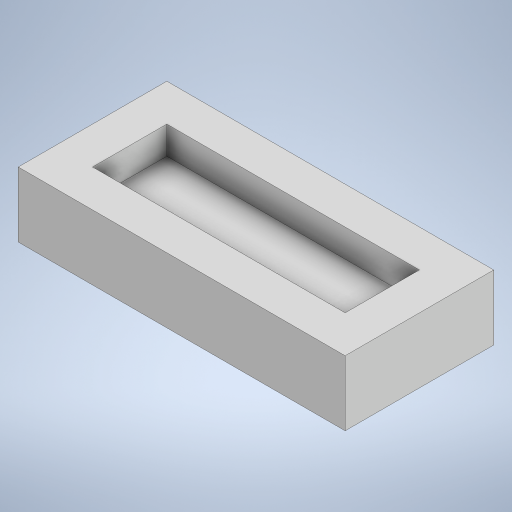
# Autodesk Inventor part: Connector Cover
Saved by Autodesk Inventor 2024 (Build 280153000, 153)
## iProperties
Created: 2023-09-15
Part Number: Connector Cover
Material: Generic
Document SubType Name: Modeling
Designer: cfang
Density: 1 g/cm^3
Appearance: Default
Author: cfang
Autodesk Inventor part; units mm, degrees
ref_plane "YZ Plane" through (0, 0, 0) normal (1, 0, 0) x (0, 1, 0)
ref_plane "XZ Plane" through (0, 0, 0) normal (0, 1, 0) x (-1, 0, 0)
ref_plane "XY Plane" through (0, 0, 0) normal (0, 0, 1) x (1, 0, 0)
sketch "Sketch1" plane through (0, 0, 0) normal (0, 1, 0) x (-1, 0, 0)
  line L0 (-8.8, -4) -> (8.8, -4)
  line L1 (8.8, -4) -> (8.8, 4)
  line L2 (8.8, 4) -> (-8.8, 4)
  line L3 (-8.8, 4) -> (-8.8, -4)
  line L4 (-8.8, -4) -> (8.8, 4) construction
  line L5 (8.8, -4) -> (-8.8, 4) construction
  point P0 (0, 0)
  dimension "d0" = 8
  dimension "d1" = 17.6
  constraints: 12 end point, 2 midpoint, 2 parallel, 1 horizontal, 1 perpendicular
  measures "d0" distance of L0.end L1.end
  measures "d1" distance of L1.end L2.end
extrude "Extrusion1" add sketch "Sketch1" along normal blind 3.5
sketch "Sketch2" plane through (0, 3.5, 0) normal (0, 1, 0) x (1, 0, 0)
  line L0 (6.8, 2) -> (-6.8, 2)
  line L1 (-6.8, 2) -> (-6.8, -2)
  line L2 (-6.8, -2) -> (6.8, -2)
  line L3 (6.8, -2) -> (6.8, 2)
  line L4 (6.8, 2) -> (-6.8, -2) construction
  line L5 (-6.8, 2) -> (6.8, -2) construction
  line L6 (-8.8, 4) -> (-8.8, -4) projected
  point P0 (0, 0)
  dimension "d4" = 4
  dimension "d5" = 2
  constraints: 12 end point, 2 midpoint, 2 parallel, 1 horizontal, 1 perpendicular
  measures "d4" distance of L0.end L1.end
  measures "d5" distance between parallel lines of L6 L1
extrude "Extrusion2" cut sketch "Sketch2" against normal blind 1.5
body "Solid1"
